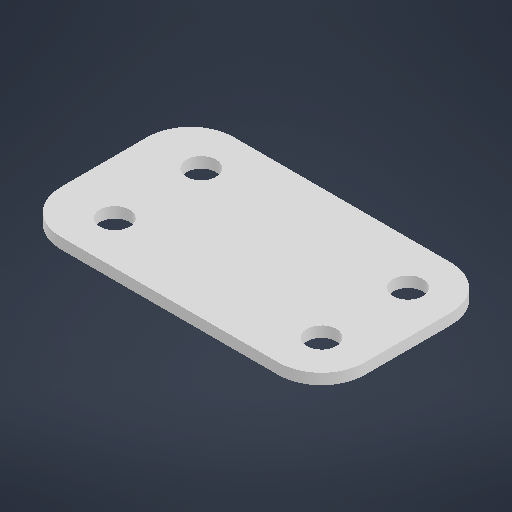
# Autodesk Inventor part: lbgrippermountpoly
Saved by Autodesk Inventor 2025.2 (Build 292293000, 293)
## iProperties
Created: 2025-04-04
Part Number: lbgrippermountpoly
Material: Generic
Document SubType Name: Modeling
Designer: Jahan
Density: 1 g/cm^3
Appearance: Default
Author: Jahan
Autodesk Inventor part; units mm, degrees
ref_plane "YZ Plane" through (0, 0, 0) normal (1, 0, 0) x (0, 1, 0)
ref_plane "XZ Plane" through (0, 0, 0) normal (0, 1, 0) x (-1, 0, 0)
ref_plane "XY Plane" through (0, 0, 0) normal (0, 0, 1) x (1, 0, 0)
sketch "Sketch1" plane through (0, 0, 0) normal (0, 1, 0) x (-1, 0, 0)
  circle A0 centre (0, 0) radius 2.1844
  circle A1 centre (30.353, 0) radius 2.1844
  line L0 (0, -12.7) -> (0, 0)
  circle A2 centre (30.353, -12.7) radius 2.1844
  circle A3 centre (0, -12.7) radius 2.1844
  circle A4 centre (0, -12.7) radius 6.35
  circle A5 centre (0, 0) radius 6.35
  line L1 (30.353, -19.05) -> (0, -19.05)
  line L2 (-6.35, -12.7) -> (-6.35, 0)
  line L3 (0, 6.35) -> (30.353, 6.35)
  line L4 (30.353, 0) -> (31.9405, 0)
  circle A6 centre (31.9405, 0) radius 6.35
  circle A7 centre (31.9405, -12.7) radius 6.35
  line L5 (30.353, 6.35) -> (31.9405, 6.35)
  line L6 (30.353, -19.05) -> (31.9405, -19.05)
  line L7 (38.2905, -12.7) -> (38.2905, 0)
  dimension "d0" = 4.3688
  dimension "d2" = 4.3688
  dimension "d4" = 4.3688
  dimension "d5" = 4.3688
  dimension "d8" = 12.7
  dimension "d9" = 12.7
  dimension "d10" = 1.5875
  dimension "d12" = 12.7
  dimension "d13" = 12.7
  constraints: 16 end point, 8 centre point, 8 point on circle, 6 coincident, 4 tangent, 1 horizontal, 1 parallel, 1 perpendicular
  measures "d0" diameter of A0
  measures "d2" diameter of A1
  measures "d4" diameter of A2
  measures "d5" diameter of A3
  measures "d8" diameter of A4
  measures "d9" diameter of A5
  measures "d10" distance of L4.start L4.end
  measures "d12" diameter of A6
  measures "d13" diameter of A7
extrude "Extrusion1" add sketch "Sketch1" along normal blind 1.5875
body "Solid1"
